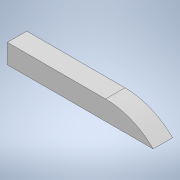
# Autodesk Inventor part: New_ThinFinger
Saved by Autodesk Inventor 2021 (Build 250183000, 183)
## iProperties
Created: 2021-08-05
Part Number: New_ThinFinger
Material: Generic
Document SubType Name: Modeling
Designer: hp
Density: 1 g/cm^3
Appearance: Default
Author: hp
Autodesk Inventor part; units mm, degrees
ref_plane "YZ Plane" through (0, 0, 0) normal (1, 0, 0) x (0, 1, 0)
ref_plane "XZ Plane" through (0, 0, 0) normal (0, 1, 0) x (-1, 0, 0)
sketch "Sketch1" plane through (0, 0, 0) normal (1, 0, 0) x (0, 1, 0)
  line L0 (-0.6, 0.6) -> (-0.6, -0.6)
  line L1 (-0.6, -0.6) -> (0.6, -0.6)
  line L2 (0.6, -0.6) -> (0.6, 0.6)
  line L3 (0.6, 0.6) -> (-0.6, 0.6)
  line L4 (-0.6, 0.6) -> (0.6, -0.6) construction
  line L5 (-0.6, -0.6) -> (0.6, 0.6) construction
  point P0 (0, 0)
  dimension "d0" = 1.2
  dimension "d1" = 1.2
  constraints: 12 end point, 2 midpoint, 2 parallel, 1 perpendicular, 1 vertical
  measures "d0" distance of L0.start L0.end
  measures "d1" distance of L1.end L0.end
extrude "Extrusion1" add sketch "Sketch1" along normal blind 9
ref_plane "Work Plane1" through (0, -0.6, 0.6) normal (0, 0, 1) x (1, 0, 0)
sketch "Sketch2" plane through (0, -0.6, 0.6) normal (0, 0, 1) x (1, 0, 0)
  line L0 (9, 0) -> (9, 1.2) projected
  line L1 (0, 1.2) -> (9, 1.2) projected
  line L2 (9, 0) -> (9, 1.2)
  line L3 (9, 1.2) -> (7.8, 1.2)
  line L4 (7.8, 1.2) -> (9, 0)
  point P0 (0, 0.6)
  dimension "d5" = 1.2
  constraints: 6 end point, 1 perpendicular, 1 point on line
  measures "d5" distance of L0.end L3.end
extrude "Extrusion2" cut sketch "Sketch2" against normal blind 9
fillet "Fillet1" radius 4.2 1 edges at (7.8, 0.6, 0)
body "Solid1"
